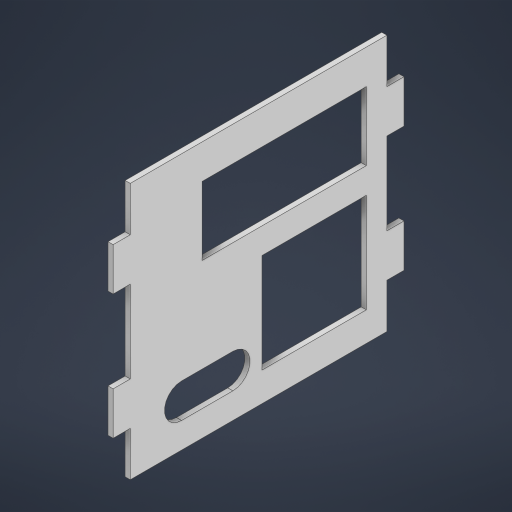
# Autodesk Inventor part: front_part
Saved by Autodesk Inventor 2023 (Build 270158000, 158)
## iProperties
Created: 2022-11-27
Part Number: front_part
Material: Generic
Document SubType Name: Modeling
Designer: washington
Density: 1 g/cm^3
Appearance: Default
Author: washington
Autodesk Inventor part; units mm, degrees
ref_plane "YZ Plane" through (0, 0, 0) normal (1, 0, 0) x (0, 1, 0)
ref_plane "XZ Plane" through (0, 0, 0) normal (0, 1, 0) x (-1, 0, 0)
ref_plane "XY Plane" through (0, 0, 0) normal (0, 0, 1) x (1, 0, 0)
sketch "Sketch1" plane through (0, 0, 0) normal (1, 0, 0) x (0, 1, 0)
  line L0 (150, 0) -> (150, -150)
  line L1 (0, -150) -> (0, 0)
  line L2 (130, -42) -> (90, -42)
  line L3 (90, -42) -> (90, -138)
  line L4 (90, -138) -> (130, -138)
  line L5 (130, -138) -> (130, -42)
  line L6 (130, -42) -> (90, -138) construction
  line L7 (90, -42) -> (130, -138) construction
  line L8 (75, -77) -> (17, -77)
  line L9 (17, -77) -> (17, -138)
  line L10 (17, -138) -> (75, -138)
  line L11 (75, -138) -> (75, -77)
  line L12 (75, -77) -> (17, -138) construction
  line L13 (17, -77) -> (75, -138) construction
  line L14 (25, -30) -> (25, -60) construction
  line L15 (35, -30) -> (35, -60)
  line L16 (15, -60) -> (15, -30)
  arc A0 (35, -30) -> (15, -30) centre (25, -30) ccw
  arc A1 (15, -60) -> (35, -60) centre (25, -60) ccw
  line L17 (124, 0) -> (124, 10)
  line L18 (124, 10) -> (99, 10)
  line L19 (99, 10) -> (99, 0)
  line L20 (51, 0) -> (51, 10)
  line L21 (51, 10) -> (26, 10)
  line L22 (26, 10) -> (26, 0)
  line L23 (150, -75) -> (168, -75)
  line L24 (124, 0) -> (150, 0)
  line L25 (0, 0) -> (26, 0)
  line L26 (51, 0) -> (99, 0)
  line L27 (124, -150) -> (124, -160)
  line L28 (124, -160) -> (99, -160)
  line L29 (99, -160) -> (99, -150)
  line L30 (51, -150) -> (51, -160)
  line L31 (51, -160) -> (26, -160)
  line L32 (26, -160) -> (26, -150)
  line L33 (150, -150) -> (124, -150)
  line L34 (99, -150) -> (51, -150)
  line L35 (26, -150) -> (0, -150)
  point P0 (110, -90)
  point P1 (46, -107.5)
  point P2 (25, -45)
  dimension "d0" = 150
  dimension "d1" = 150
  dimension "d2" = 90
  dimension "d3" = 110
  dimension "d4" = 40
  dimension "d5" = 96
  dimension "d6" = 58
  dimension "d7" = 61
  dimension "d8" = 46
  dimension "d9" = 96
  dimension "d10" = 25
  dimension "d11" = 30
  dimension "d12" = 30
  dimension "d13" = 10
  dimension "d16" = 25
  dimension "d17" = 10
  dimension "d18" = 26
  dimension "d19" = 10
  dimension "d20" = 25
  dimension "d21" = 26
  dimension "d24" = 33
  dimension "d25" = 75
  dimension "d26" = 18
  constraints: 74 end point, 15 parallel, 13 perpendicular, 8 symmetric about line, 6 horizontal, 6 midpoint, 4 point on circle, 4 tangent, 3 vertical, 2 centre point
  measures "d0" distance of L0.start L0.end
  measures "d1" distance of L0.end L1.start
  measures "d2" vertical distance of point (110, -90) L1.end
  measures "d3" horizontal distance of point (110, -90) L1.end
  measures "d4" distance of L3.end L4.end
  measures "d5" distance of L2.end L3.end
  measures "d6" distance of L9.end L10.end
  measures "d7" distance of L8.end L9.end
  measures "d8" horizontal distance of point (46, -107.5) L1.end
  measures "d9" distance between parallel lines of L2 L10
  measures "d10" horizontal distance of point (25, -45) L1.end
  measures "d11" vertical distance of L14.start L1.end
  measures "d12" distance of L14.end L14.start
  measures "d13" radius of A0
  measures "d16" distance of L17.end L18.end
  measures "d17" distance of L17.start L17.end
  measures "d18" distance between parallel lines of L0 L17
  measures "d19" distance of L20.start L20.end
  measures "d20" distance of L20.end L21.end
  measures "d21" distance from line of L22 L1.end
  measures "d24" distance between parallel lines of L23 L2
  measures "d25" distance between parallel lines of L23 L26
  measures "d26" distance from line of L23.end L0
extrude "Extrusion1" add sketch "Sketch1" along normal blind 3
body "Solid1"
